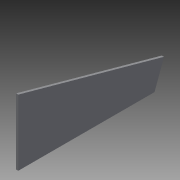
# Autodesk Inventor part: sponda laterale policarbonato
Saved by Autodesk Inventor 2014 SP2 (Build 180246200, 246)
## iProperties
Created: 2019-04-11
Part Number: sponda laterale policarbonato
Material: Generic
Document SubType Name: Modeling
Designer: GauchoHP
Density: 1 g/cm^3
Appearance: Default
Author: GauchoHP
Autodesk Inventor part; units mm, degrees
ref_plane "YZ Plane" through (0, 0, 0) normal (1, 0, 0) x (0, 1, 0)
ref_plane "XZ Plane" through (0, 0, 0) normal (0, 1, 0) x (-1, 0, 0)
ref_plane "XY Plane" through (0, 0, 0) normal (0, 0, 1) x (1, 0, 0)
sketch "Sketch1" plane through (0, 0, 0) normal (1, 0, 0) x (0, 1, 0)
  line L0 (104.552, -76.3353) -> (-138.448, -76.3353)
  line L1 (-138.448, -76.3353) -> (-138.448, 38.6647)
  line L2 (-138.448, 38.6647) -> (118.8782, -29.4764)
  line L3 (104.552, -76.3353) -> (118.8782, -29.4764)
  point P0 (0, 0)
  dimension "d7" = 90
  dimension "d8" = 243
  dimension "d9" = 107
  dimension "d10" = 49
  dimension "d11" = 115
  constraints: 8 end point, 1 horizontal
  measures "d7" angle of L1 L0
  measures "d8" distance of L0.start L0.end
  measures "d9" angle of L0 L3
  measures "d10" distance of L0.start L2.end
  measures "d11" distance of L0.end L1.end
extrude "Extrusion1" add sketch "Sketch1" along normal blind 4
body "Solid1"
